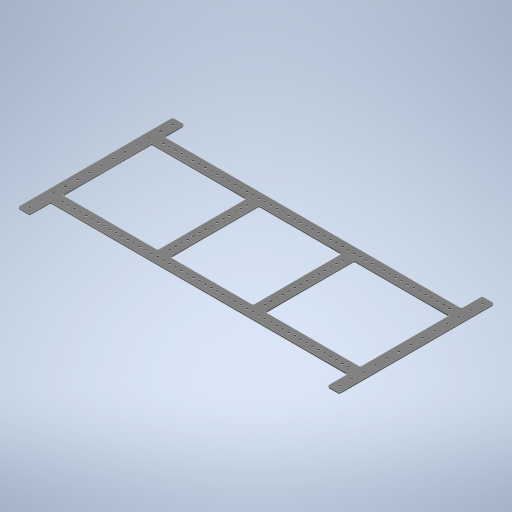
# Autodesk Inventor part: 27in_2_0 H_support
Saved by Autodesk Inventor 2023 (Build 270158000, 158)
## iProperties
Created: 2023-11-06
Part Number: 27in_2_0 H_support
Material: Aluminum 6061
Document SubType Name: Modeling
Designer: robotics
Density: 2.7 g/cm^3
Appearance: Smooth - Black
Mass: 477.924 g
Surface Area: 1334.04 cm^2
Volume: 177.009 cm^3
Author: robotics
Autodesk Inventor part; units mm, degrees
ref_plane "YZ Plane" through (0, 0, 0) normal (1, 0, 0) x (0, 1, 0)
ref_plane "XZ Plane" through (0, 0, 0) normal (0, 1, 0) x (-1, 0, 0)
ref_plane "XY Plane" through (0, 0, 0) normal (0, 0, 1) x (1, 0, 0)
sketch "Sketch1" plane through (0, 0, 0) normal (0, 1, 0) x (-1, 0, 0)
  line L0 (0, 0) -> (0, -330.2)
  line L1 (0, -330.2) -> (-25.4, -330.2)
  line L2 (-25.4, -330.2) -> (-25.4, -285.75)
  line L3 (-25.4, -285.75) -> (-660.4, -285.75)
  line L4 (-660.4, -285.75) -> (-660.4, -330.2)
  line L5 (-660.4, -330.2) -> (-685.8, -330.2)
  line L6 (-685.8, -330.2) -> (-685.8, 0)
  line L7 (-685.8, 0) -> (-660.4, 0)
  line L8 (-660.4, 0) -> (-660.4, -44.45)
  line L9 (-660.4, -44.45) -> (-25.4, -44.45)
  line L10 (-25.4, -44.45) -> (-25.4, 0)
  line L11 (-25.4, 0) -> (0, 0)
  line L12 (-25.4, -69.85) -> (-228.6, -69.85)
  line L13 (-228.6, -69.85) -> (-228.6, -260.35)
  line L14 (-228.6, -260.35) -> (-25.4, -260.35)
  line L15 (-25.4, -260.35) -> (-25.4, -69.85)
  line L16 (-254, -69.85) -> (-431.8, -69.85)
  line L17 (-431.8, -69.85) -> (-431.8, -260.35)
  line L18 (-431.8, -260.35) -> (-254, -260.35)
  line L19 (-254, -260.35) -> (-254, -69.85)
  line L20 (-457.2, -69.85) -> (-660.4, -69.85)
  line L21 (-660.4, -69.85) -> (-660.4, -260.35)
  line L22 (-660.4, -260.35) -> (-457.2, -260.35)
  line L23 (-457.2, -260.35) -> (-457.2, -69.85)
  circle A0 centre (-12.7, -12.7) radius 2.8067
  circle A1 centre (-12.7, -38.1) radius 2.8067
  circle A2 centre (-12.7, -63.5) radius 2.8067
  circle A3 centre (-12.7, -88.9) radius 2.8067
  circle A4 centre (-12.7, -114.3) radius 2.8067
  circle A5 centre (-12.7, -139.7) radius 2.8067
  circle A6 centre (-12.7, -165.1) radius 2.8067
  circle A7 centre (-12.7, -190.5) radius 2.8067
  circle A8 centre (-12.7, -215.9) radius 2.8067
  circle A9 centre (-12.7, -241.3) radius 2.8067
  circle A10 centre (-12.7, -266.7) radius 2.8067
  circle A11 centre (-12.7, -292.1) radius 2.8067
  circle A12 centre (-12.7, -317.5) radius 2.8067
  line L24 (-342.9, -69.85) -> (-342.9, -260.35) construction
  line L25 (-342.9, -165.1) -> (-25.4, -165.1) construction
  circle A13 centre (-38.1, -57.15) radius 2.8067
  circle A14 centre (-50.8, -57.15) radius 2.8067
  circle A15 centre (-63.5, -57.15) radius 2.8067
  circle A16 centre (-76.2, -57.15) radius 2.8067
  circle A17 centre (-88.9, -57.15) radius 2.8067
  circle A18 centre (-101.6, -57.15) radius 2.8067
  circle A19 centre (-114.3, -57.15) radius 2.8067
  circle A20 centre (-127, -57.15) radius 2.8067
  circle A21 centre (-139.7, -57.15) radius 2.8067
  circle A22 centre (-152.4, -57.15) radius 2.8067
  circle A23 centre (-165.1, -57.15) radius 2.8067
  circle A24 centre (-177.8, -57.15) radius 2.8067
  circle A25 centre (-190.5, -57.15) radius 2.8067
  circle A26 centre (-203.2, -57.15) radius 2.8067
  circle A27 centre (-215.9, -57.15) radius 2.8067
  circle A28 centre (-228.6, -57.15) radius 2.8067
  circle A29 centre (-241.3, -57.15) radius 2.8067
  circle A30 centre (-254, -57.15) radius 2.8067
  circle A31 centre (-266.7, -57.15) radius 2.8067
  circle A32 centre (-279.4, -57.15) radius 2.8067
  circle A33 centre (-292.1, -57.15) radius 2.8067
  circle A34 centre (-304.8, -57.15) radius 2.8067
  circle A35 centre (-317.5, -57.15) radius 2.8067
  circle A36 centre (-330.2, -57.15) radius 2.8067
  circle A37 centre (-342.9, -57.15) radius 2.8067
  circle A38 centre (-355.6, -57.15) radius 2.8067
  circle A39 centre (-368.3, -57.15) radius 2.8067
  circle A40 centre (-381, -57.15) radius 2.8067
  circle A41 centre (-393.7, -57.15) radius 2.8067
  circle A42 centre (-406.4, -57.15) radius 2.8067
  circle A43 centre (-419.1, -57.15) radius 2.8067
  circle A44 centre (-431.8, -57.15) radius 2.8067
  circle A45 centre (-444.5, -57.15) radius 2.8067
  circle A46 centre (-457.2, -57.15) radius 2.8067
  circle A47 centre (-469.9, -57.15) radius 2.8067
  circle A48 centre (-482.6, -57.15) radius 2.8067
  circle A49 centre (-495.3, -57.15) radius 2.8067
  circle A50 centre (-508, -57.15) radius 2.8067
  circle A51 centre (-520.7, -57.15) radius 2.8067
  circle A52 centre (-533.4, -57.15) radius 2.8067
  circle A53 centre (-546.1, -57.15) radius 2.8067
  circle A54 centre (-558.8, -57.15) radius 2.8067
  circle A55 centre (-571.5, -57.15) radius 2.8067
  circle A56 centre (-584.2, -57.15) radius 2.8067
  circle A57 centre (-596.9, -57.15) radius 2.8067
  circle A58 centre (-609.6, -57.15) radius 2.8067
  circle A59 centre (-622.3, -57.15) radius 2.8067
  circle A60 centre (-635, -57.15) radius 2.8067
  circle A61 centre (-647.7, -57.15) radius 2.8067
  circle A62 centre (-241.3, -82.55) radius 2.8067
  circle A63 centre (-241.3, -95.25) radius 2.8067
  circle A64 centre (-241.3, -107.95) radius 2.8067
  circle A65 centre (-241.3, -120.65) radius 2.8067
  circle A66 centre (-241.3, -133.35) radius 2.8067
  circle A67 centre (-241.3, -146.05) radius 2.8067
  circle A68 centre (-241.3, -158.75) radius 2.8067
  circle A69 centre (-241.3, -171.45) radius 2.8067
  circle A70 centre (-241.3, -184.15) radius 2.8067
  circle A71 centre (-241.3, -196.85) radius 2.8067
  circle A72 centre (-241.3, -209.55) radius 2.8067
  circle A73 centre (-241.3, -222.25) radius 2.8067
  circle A74 centre (-241.3, -234.95) radius 2.8067
  circle A75 centre (-241.3, -247.65) radius 2.8067
  circle A76 centre (-673.1, -12.7) radius 2.8067
  circle A77 centre (-673.1, -38.1) radius 2.8067
  circle A78 centre (-673.1, -63.5) radius 2.8067
  circle A79 centre (-673.1, -88.9) radius 2.8067
  circle A80 centre (-673.1, -114.3) radius 2.8067
  circle A81 centre (-673.1, -139.7) radius 2.8067
  circle A82 centre (-673.1, -165.1) radius 2.8067
  circle A83 centre (-673.1, -190.5) radius 2.8067
  circle A84 centre (-673.1, -215.9) radius 2.8067
  circle A85 centre (-673.1, -241.3) radius 2.8067
  circle A86 centre (-673.1, -266.7) radius 2.8067
  circle A87 centre (-673.1, -292.1) radius 2.8067
  circle A88 centre (-673.1, -317.5) radius 2.8067
  circle A89 centre (-444.5, -82.55) radius 2.8067
  circle A90 centre (-444.5, -95.25) radius 2.8067
  circle A91 centre (-444.5, -107.95) radius 2.8067
  circle A92 centre (-444.5, -120.65) radius 2.8067
  circle A93 centre (-444.5, -133.35) radius 2.8067
  circle A94 centre (-444.5, -146.05) radius 2.8067
  circle A95 centre (-444.5, -158.75) radius 2.8067
  circle A96 centre (-444.5, -171.45) radius 2.8067
  circle A97 centre (-444.5, -184.15) radius 2.8067
  circle A98 centre (-444.5, -196.85) radius 2.8067
  circle A99 centre (-444.5, -209.55) radius 2.8067
  circle A100 centre (-444.5, -222.25) radius 2.8067
  circle A101 centre (-444.5, -234.95) radius 2.8067
  circle A102 centre (-444.5, -247.65) radius 2.8067
  circle A103 centre (-38.1, -273.05) radius 2.8067
  circle A104 centre (-50.8, -273.05) radius 2.8067
  circle A105 centre (-63.5, -273.05) radius 2.8067
  circle A106 centre (-76.2, -273.05) radius 2.8067
  circle A107 centre (-88.9, -273.05) radius 2.8067
  circle A108 centre (-101.6, -273.05) radius 2.8067
  circle A109 centre (-114.3, -273.05) radius 2.8067
  circle A110 centre (-127, -273.05) radius 2.8067
  circle A111 centre (-139.7, -273.05) radius 2.8067
  circle A112 centre (-152.4, -273.05) radius 2.8067
  circle A113 centre (-165.1, -273.05) radius 2.8067
  circle A114 centre (-177.8, -273.05) radius 2.8067
  circle A115 centre (-190.5, -273.05) radius 2.8067
  circle A116 centre (-203.2, -273.05) radius 2.8067
  circle A117 centre (-215.9, -273.05) radius 2.8067
  circle A118 centre (-228.6, -273.05) radius 2.8067
  circle A119 centre (-241.3, -273.05) radius 2.8067
  circle A120 centre (-254, -273.05) radius 2.8067
  circle A121 centre (-266.7, -273.05) radius 2.8067
  circle A122 centre (-279.4, -273.05) radius 2.8067
  circle A123 centre (-292.1, -273.05) radius 2.8067
  circle A124 centre (-304.8, -273.05) radius 2.8067
  circle A125 centre (-317.5, -273.05) radius 2.8067
  circle A126 centre (-330.2, -273.05) radius 2.8067
  circle A127 centre (-342.9, -273.05) radius 2.8067
  circle A128 centre (-355.6, -273.05) radius 2.8067
  circle A129 centre (-368.3, -273.05) radius 2.8067
  circle A130 centre (-381, -273.05) radius 2.8067
  circle A131 centre (-393.7, -273.05) radius 2.8067
  circle A132 centre (-406.4, -273.05) radius 2.8067
  circle A133 centre (-419.1, -273.05) radius 2.8067
  circle A134 centre (-431.8, -273.05) radius 2.8067
  circle A135 centre (-444.5, -273.05) radius 2.8067
  circle A136 centre (-457.2, -273.05) radius 2.8067
  circle A137 centre (-469.9, -273.05) radius 2.8067
  circle A138 centre (-482.6, -273.05) radius 2.8067
  circle A139 centre (-495.3, -273.05) radius 2.8067
  circle A140 centre (-508, -273.05) radius 2.8067
  circle A141 centre (-520.7, -273.05) radius 2.8067
  circle A142 centre (-533.4, -273.05) radius 2.8067
  circle A143 centre (-546.1, -273.05) radius 2.8067
  circle A144 centre (-558.8, -273.05) radius 2.8067
  circle A145 centre (-571.5, -273.05) radius 2.8067
  circle A146 centre (-584.2, -273.05) radius 2.8067
  circle A147 centre (-596.9, -273.05) radius 2.8067
  circle A148 centre (-609.6, -273.05) radius 2.8067
  circle A149 centre (-622.3, -273.05) radius 2.8067
  circle A150 centre (-635, -273.05) radius 2.8067
  circle A151 centre (-647.7, -273.05) radius 2.8067
  dimension "d0" = 25.4
  dimension "d1" = 25.4
  dimension "d2" = 25.4
  dimension "d3" = 25.4
  dimension "d4" = 25.4
  dimension "d5" = 25.4
  dimension "d6" = 203.2
  dimension "d7" = 203.2
  dimension "d8" = 685.8
  dimension "d9" = 190.5
  dimension "d10" = 330.2
  dimension "d11" = 12.7
  dimension "d12" = 12.7
  dimension "d13" = 5.6134
  dimension "d16" = 25.4
  dimension "d21" = 12.7
  dimension "d22" = 12.7
  dimension "d25" = 12.7
  dimension "d30" = 12.7
  dimension "d31" = 12.7
  dimension "d34" = 12.7
  constraints: 152 centre point, 76 symmetric about line, 52 end point, 12 perpendicular, 10 point on line, 6 parallel, 4 horizontal, 4 horizontal alignment, 4 midpoint, 3 vertical, 2 equal length, 2 equal radius, 2 vertical alignment, 1 coincident, 222 other
  measures "d0" distance of L6.end L7.end
  measures "d1" distance of L10.end L0.start
  measures "d2" distance between parallel lines of L14 L3
  measures "d3" distance between parallel lines of L9 L12
  measures "d4" distance between parallel lines of L19 L13
  measures "d5" distance between parallel lines of L23 L17
  measures "d6" distance from line of L25.end L13
  measures "d7" distance between parallel lines of L21 L23
  measures "d8" distance between parallel lines of L6 L0
  measures "d9" distance between parallel lines of L12 L14
  measures "d10" distance of L0.start L0.end
  measures "d11" distance from line of A0.centre L0
  measures "d12" distance from line of A0.centre L11
  measures "d13" diameter of A0
  measures "d16" distance of A0.centre A1.centre
  measures "d21" distance from line of A13.centre L12
  measures "d22" horizontal distance of A13.centre L12.start
  measures "d25" distance of A13.centre A14.centre
  measures "d30" horizontal distance of A62.centre L12.end
  measures "d31" distance from line of L13 A62.centre
  measures "d34" distance of A62.centre A63.centre
extrude "Extrusion1" add sketch "Sketch1" along normal blind 3.175
fillet "Fillet1" radius 3.175 24 edges at (25.4, 1.5875, -260.35) (25.4, 1.5875, -69.85) (228.6, 1.5875, -69.85) (228.6, 1.5875, -260.35) (25.4, 1.5875, -285.75) (25.4, 1.5875, -44.45) (254, 1.5875, -260.35) (254, 1.5875, -69.85) (431.8, 1.5875, -69.85) (431.8, 1.5875, -260.35) (457.2, 1.5875, -69.85) (660.4, 1.5875, -69.85) (660.4, 1.5875, -260.35) (457.2, 1.5875, -260.35) (660.4, 1.5875, -285.75) (660.4, 1.5875, -44.45) (660.4, 1.5875, 0) (685.8, 1.5875, 0) (685.8, 1.5875, -330.2) (660.4, 1.5875, -330.2) (0, 1.5875, -330.2) (25.4, 1.5875, -330.2) (0, 1.5875, 0) (25.4, 1.5875, 0)
body "Solid1"
